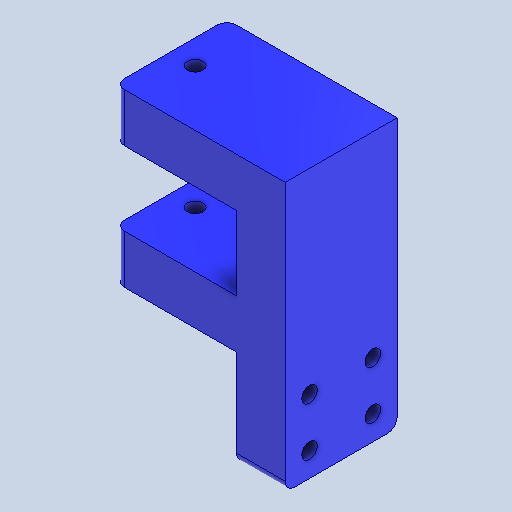
# Autodesk Inventor part: dribl-v1-3DP-cc-f-1
Saved by Autodesk Inventor 2025.2 (Build 292293000, 293)
## iProperties
Created: 2025-03-16
Part Number: dribl-v1-3DP-cc-f-1
Material: ABS プラスチック
Document SubType Name: Modeling
Designer: haruy
Density: 1.06 g/cm^3
Appearance: 青 - 壁塗料 - 光沢
Author: haruy
Autodesk Inventor part; units mm, degrees
ref_plane "YZ Plane" through (0, 0, 0) normal (1, 0, 0) x (0, 1, 0)
ref_plane "XZ Plane" through (0, 0, 0) normal (0, 1, 0) x (-1, 0, 0)
ref_plane "XY Plane" through (0, 0, 0) normal (0, 0, 1) x (1, 0, 0)
sketch "スケッチ1" plane through (0, 0, 0) normal (1, 0, 0) x (0, 1, 0)
  line L0 (0, 0) -> (15.2, 0)
  line L1 (15.2, 0) -> (15.2, -62.0281)
  line L2 (15.2, -62.0281) -> (0, -62.0281)
  line L3 (0, -62.0281) -> (0, 0)
  circle A0 centre (-15, -24.3937) radius 1.6
  circle A1 centre (-25, -24.3937) radius 1.6
  circle A2 centre (-15, -37.3937) radius 1.6
  circle A3 centre (-25, -37.3937) radius 1.6
  line L4 (25.2, -19.3937) -> (-10, -19.3937)
  line L5 (-10, -19.3937) -> (-10, -42.3937)
  line L6 (-10, -42.3937) -> (25.2, -42.3937)
  line L7 (25.2, -42.3937) -> (25.2, -19.3937)
  line L8 (-10, -19.3937) -> (-30, -19.3937)
  line L9 (-30, -19.3937) -> (-30, -42.3937)
  line L10 (-30, -42.3937) -> (-10, -42.3937)
  line L11 (-10, -42.3937) -> (-10, -19.3937)
  point P0 (0, -42.3937)
  point P1 (0, -19.3937)
  point P2 (15.2, -19.3937)
  point P3 (15.2, -42.3937)
  point P4 (-10, -42.3937)
  dimension "d0" = 15.2
  dimension "d1" = 3.2
  dimension "d2" = 3.2
  dimension "d3" = 3.2
  dimension "d4" = 3.2
  dimension "d5" = 10
  dimension "d6" = 10
  dimension "d7" = 13
  dimension "d8" = 13
  dimension "d9" = 0
  dimension "d10" = 0
  dimension "d12" = 10
  dimension "d13" = 10
  dimension "d14" = 5
  dimension "d15" = 5
  dimension "d16" = 5
  dimension "d17" = 0
  dimension "d18" = 5
  constraints: 24 end point, 6 parallel, 4 centre point, 3 horizontal, 3 perpendicular
  measures "d0" distance of L1.end L2.end
  measures "d1" diameter of A0
  measures "d2" diameter of A1
  measures "d3" diameter of A2
  measures "d4" diameter of A3
  measures "d5" distance of A1.centre A0.centre
  measures "d6" distance of A3.centre A2.centre
  measures "d7" distance of A2.centre A0.centre
  measures "d8" distance of A3.centre A1.centre
  measures "d9" vertical distance of A1.centre A0.centre
  measures "d10" horizontal distance of A0.centre A2.centre
  measures "d12" distance between parallel lines of L5 L3
  measures "d13" distance between parallel lines of L7 L1
  measures "d14" distance from line of A0.centre L5
  measures "d15" distance from line of L4 A0.centre
  measures "d16" distance from line of L6 A2.centre
  measures "d17" distance between parallel lines of L6 L10
  measures "d18" distance from line of L9 A1.centre
extrude "押し出し1" add sketch "スケッチ1" against normal blind 25 contours L3 L6 L5 L4 | L4 L7 L6 L1
extrude "押し出し2" add sketch "スケッチ1" along normal blind 10 contours L4 L1 L6 L3 | L3 L6 L5 L4 | L4 L7 L6 L1 | L5 L10 L9 L8
sketch "スケッチ2" plane through (-25, 25.2, -19.3937) normal (0, 1, 0) x (1, 0, 0)
  line L0 (25, 23) -> (0, 23) projected
  line L1 (5, 23) -> (5, 0)
  line L2 (25, 0) -> (0, 0) projected
  line L3 (0, 0) -> (0, 23) projected
  point P0 (25, -19.3937)
  point P1 (5, 11.5)
  dimension "d23" = 5
  constraints: 2 end point, 2 point on line, 1 midpoint, 1 vertical
  measures "d23" distance between parallel lines of L1 L3
hole "穴1" at (-20, 25.2, -30.8937) direction (0, -1, 0) diameter 3.2 end through all
fillet "フィレット1" radius 2 6 edges at (-25, 20.2, -19.3937) (-25, -5, -19.3937) (-25, -5, -42.3937) (-25, 20.2, -42.3937) (5, -30, -19.3937) (5, -30, -42.3937)
equation "\"d6\" = d5"
equation "\"d8\" = d7"
